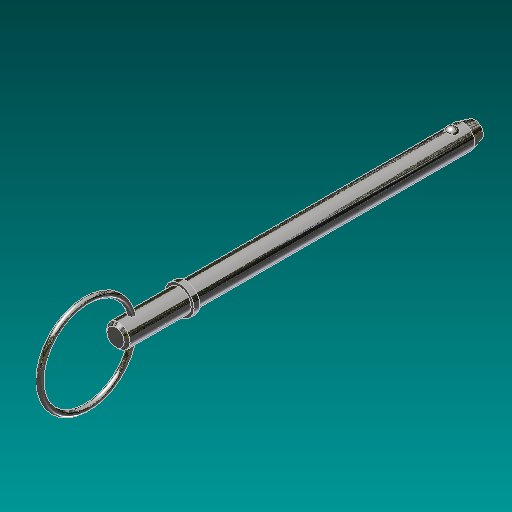
# Autodesk Inventor part: Quick release pin
Saved by Autodesk Inventor 2017 (Build 210142000, 142)
## iProperties
Created: 2018-06-13
Part Number: Quick release pin
Material: Stainless Steel
Document SubType Name: Modeling
Designer: Graeme_Van_Dongen
Density: 8 g/cm^3
Appearance: Semi-Polished
Description: Ø1/4" x 2.8" QUICK RELEASE PIN, STAINLESS, SPAENAUR #233-974
Author: Graeme_Van_Dongen
Autodesk Inventor part; units mm, degrees
ref_plane "YZ Plane" through (0, 0, 0) normal (1, 0, 0) x (0, 1, 0)
ref_plane "XZ Plane" through (0, 0, 0) normal (0, 1, 0) x (-1, 0, 0)
ref_plane "XY Plane" through (0, 0, 0) normal (0, 0, 1) x (1, 0, 0)
sketch "Sketch1" plane through (0, 0, 0) normal (0, 0, 1) x (1, 0, 0)
  circle A0 centre (0, 0) radius 3.175
  dimension "d0" = 6.35
  constraints: 1 centre point, 1 coincident
  measures "d0" diameter of A0
extrude "Extrusion1" add sketch "Sketch1" along normal blind 19.05 and the other way blind 79.0575
sketch "Sketch2" plane through (0, 0, 0) normal (0, 0, 1) x (1, 0, 0)
  circle A0 centre (0, 0) radius 3.9688
  dimension "d5" = 7.9375
  constraints: 1 centre point, 1 coincident
  measures "d5" diameter of A0
extrude "Extrusion2" add sketch "Sketch2" along normal blind 1.5875
chamfer "Chamfer1" distance 3.175 angle 15 1 edges at (-3.175, 0, -79.0575) measured on face at (-3.175, 0, -78.5575)
chamfer "Chamfer2" distance 0.7937 angle 45 1 edges at (-3.175, 0, 19.05)
sketch "Sketch3" plane through (0, 0, 0) normal (1, 0, 0) x (0, 1, 0)
  line L0 (0, -72.7075) -> (4.064, -72.7075)
  arc A0 (4.064, -72.7075) -> (2.4765, -71.12) centre (2.4765, -72.7075) ccw
  line L1 (2.4765, -71.12) -> (0, -71.12)
  line L2 (0, -71.12) -> (0, -72.7075)
  point P0 (0, 0)
  dimension "d14" = 3.175
  dimension "d15" = 71.12
  dimension "d16" = 4.064
  constraints: 6 end point, 2 point on circle, 2 point on line, 1 centre point, 1 horizontal, 1 parallel, 1 perpendicular, 1 tangent
  measures "d14" diameter of L1 L0
  measures "d15" distance from line of point (0, 0) L1
  measures "d16" distance of L0.start L0.end
revolve "Revolution1" add sketch "Sketch3" angle 360 about axis through (0, 0, -72.7075) along (0, 1, 0)
sketch "Sketch4" plane through (0, 0, 0) normal (1, 0, 0) x (0, 1, 0)
  circle A0 centre (0, 26.9875) radius 12.7
  point P0 (0, 0)
  dimension "d18" = 25.4
  dimension "d19" = 26.9875
  constraints: 1 centre point, 1 vertical alignment
  measures "d18" diameter of A0
  measures "d19" distance of point (0, 0) A0.centre
sketch "Sketch5" plane through (0, 0, 0) normal (0, 1, 0) x (-1, 0, 0)
  line L0 (0, 39.6875) -> (0, 14.2875) construction
  circle A0 centre (0, 39.6875) radius 0.7937
  point P0 (0, 0)
  dimension "d20" = 1.5875
  constraints: 1 centre point, 1 coincident
  measures "d20" diameter of A0
sweep "Sweep1" add profiles "Sketch5" path "Sketch4"
body "Solid1"
